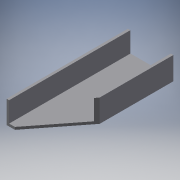
# Autodesk Inventor part: Horizontal channel right
Saved by Autodesk Inventor 2016 (Build 200138000, 138)
## iProperties
Created: 2015-02-04
Part Number: Horizontal channel right
Material: Generic
Document SubType Name: Modeling
Designer: degan
Density: 1 g/cm^3
Appearance: Default
Author: degan
Autodesk Inventor part; units mm, degrees
ref_plane "YZ Plane" through (0, 0, 0) normal (1, 0, 0) x (0, 1, 0)
ref_plane "XZ Plane" through (0, 0, 0) normal (0, 1, 0) x (-1, 0, 0)
ref_plane "XY Plane" through (0, 0, 0) normal (0, 0, 1) x (1, 0, 0)
sketch "Sketch1" plane through (0, 0, 0) normal (0, 0, 1) x (1, 0, 0)
  line L0 (24.1101, 28.575) -> (24.1101, 0)
  line L1 (24.1101, 0) -> (-33.0399, 0)
  line L2 (-33.0399, 0) -> (-33.0399, 28.575)
  line L3 (-29.8649, 28.575) -> (-29.8649, 3.175)
  line L4 (-29.8649, 3.175) -> (20.9351, 3.175)
  line L5 (20.9351, 3.175) -> (20.9351, 28.575)
  line L6 (-33.0399, 28.575) -> (-29.8649, 28.575)
  line L7 (24.1101, 28.575) -> (20.9351, 28.575)
  point P0 (0, 0)
  dimension "d0" = 57.15
  dimension "d1" = 28.575
  dimension "d2" = 3.175
  dimension "d18" = 28.575
  constraints: 16 end point, 3 equal length, 1 perpendicular, 2 other
  measures "d0" distance of L0.end L1.end
  measures "d1" distance of L1.end L2.end
  measures "d2" distance between parallel lines of L0 L5
  measures "d18" distance of L0.start L0.end
extrude "Extrusion1" add sketch "Sketch1" against normal blind 152.4
sketch "Sketch5" plane through (-33.0399, 0, 0) normal (0, -1, 0) x (1, 0, 0)
  line L0 (0, 0) -> (57.15, 0) projected
  line L1 (57.15, 0) -> (57.15, -152.4) projected
  line L2 (57.15, -152.4) -> (57.15, -59.69)
  line L3 (57.15, 0) -> (57.15, -152.4) projected
  line L4 (57.15, -59.69) -> (10.5151, 0)
  line L5 (10.5151, 0) -> (57.15, 0)
  line L6 (57.15, 0) -> (57.15, -59.69)
  point P0 (33.0399, 0)
  dimension "d14" = 92.71
  dimension "d15" = 38
  constraints: 8 end point, 2 point on line, 1 collinear, 1 perpendicular
  measures "d14" distance of L1.end L2.end
  measures "d15" angle of L4 L1
extrude "Extrusion4" cut sketch "Sketch5" against normal through all
body "Solid1"
